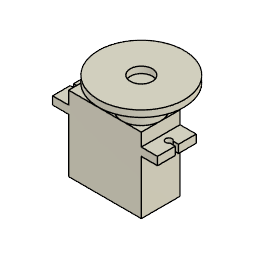
Enclosure (Autodesk Fusion 360 archive; units mm, degrees)
design "Servo"
Autodesk Fusion 360 part; units mm, degrees
sketch "Sketch1" plane through (0, 0, 0) normal (0, 0, 1) x (1, 0, 0)
  line L0 (0, 0) -> (22.5, 0)
  line L1 (22.5, 23.2) -> (0, 23.2)
  line L2 (22.5, 23.2) -> (22.5, 19.2)
  line L3 (22.5, 19.2) -> (27.5, 19.2)
  line L4 (27.5, 19.2) -> (27.5, 16.7)
  line L5 (27.5, 16.7) -> (22.5, 16.7)
  line L6 (0, 23.2) -> (0, 19.2)
  line L7 (0, 19.2) -> (-5, 19.2)
  line L8 (-5, 19.2) -> (-5, 16.7)
  line L9 (-5, 16.7) -> (0, 16.7)
  line L10 (22.5, 0) -> (22.5, 16.7)
  line L11 (22.5, 19.2) -> (22.5, 23.2)
  line L12 (0, 23.2) -> (0, 19.2)
  line L13 (0, 16.7) -> (0, 0)
  dimension "d1" = 22.5
  dimension "d2" = 23.2
  dimension "d3" = 4
  dimension "d4" = 5
  dimension "d5" = 2.5
  dimension "d6" = 4
  dimension "d7" = 5
  dimension "d8" = 2.5
  constraint coincident L0.start L13.end
  constraint horizontal L0
  constraint perpendicular L0 L10
  constraint perpendicular L1 L11
  constraint perpendicular L0 L13
  constraint perpendicular L1 L2
  constraint perpendicular L2 L3
  constraint perpendicular L3 L4
  constraint perpendicular L5 L10
  constraint perpendicular L1 L6
  constraint perpendicular L6 L7
  constraint perpendicular L7 L8
  constraint perpendicular L9 L13
  constraint collinear L10 L11
  constraint collinear L12 L13
  measures "d1" distance of L0.start L0.end
  measures "d2" distance of L0.end L1.start
  measures "d3" distance of L1.start L2.end
  measures "d4" distance of L2.end L3.end
  measures "d5" distance of L3.end L4.end
  measures "d6" distance of L1.end L6.end
  measures "d7" distance of L6.end L7.end
  measures "d8" distance of L7.end L8.end
extrude "Extrude1" add sketch "Sketch1" along normal blind 12
move_body "Move1" bodies 1 to x (1, 0, 0) y (0, 0, 1) z (0, -1, 0) at (0, 35.2, 8.8)
sketch "Sketch2" plane through (0, 0, 28) normal (0, 0, 1) x (-1, 0, 0)
  line L0 (-27.5, -35.2) -> (-22.5, -35.2)
  line L1 (-22.5, -35.2) -> (-22.5, -23.2)
  line L2 (-22.5, -23.2) -> (-27.5, -23.2)
  line L3 (-27.5, -23.2) -> (-27.5, -35.2)
  line L4 (-27.5, -29.2) -> (-27.5, -29.7)
  line L5 (-27.5, -29.2) -> (-27.5, -28.7)
  line L6 (-27.5, -29.7) -> (-25.866, -29.7)
  line L7 (-27.5, -28.7) -> (-25.866, -28.7)
  arc A0 (-25.866, -29.7) -> (-25.866, -28.7) centre (-25, -29.2) ccw
  dimension "d11" = 2
  dimension "d12" = 0.5
  dimension "d13" = 0.5
  constraint midpoint L3 L4.start
  constraint coincident L3 L4.end
  constraint coincident L3 L5.end
  constraint perpendicular L4 L6
  constraint perpendicular L5 L7
  measures "d11" diameter of A0
  measures "d12" distance of L4.start L4.end
  measures "d13" distance of L4.start L5.end
extrude "Extrude2" cut sketch "Sketch2" against normal blind 7 contours L3 L4 L5 L6 L7 A0
sketch "Sketch3" plane through (0, 0, 28) normal (0, 0, 1) x (-1, 0, 0)
  line L0 (0, -35.2) -> (5, -35.2)
  line L1 (5, -35.2) -> (5, -23.2)
  line L2 (5, -23.2) -> (0, -23.2)
  line L3 (0, -23.2) -> (0, -35.2)
  line L4 (0, -29.2) -> (1.5, -29.2)
  line L5 (5, -29.2) -> (5, -29.7)
  line L6 (5, -29.2) -> (5, -28.7)
  line L7 (5, -29.7) -> (3.366, -29.7)
  line L8 (5, -28.7) -> (3.366, -28.7)
  arc A0 (3.366, -28.7) -> (3.366, -29.7) centre (2.5, -29.2) ccw
  dimension "d16" = 1.5
  dimension "d17" = 2
  dimension "d18" = 0.5
  dimension "d19" = 0.5
  constraint midpoint L3 L4.start
  constraint perpendicular L3 L4
  constraint coincident L4.end A0
  constraint midpoint L1 L5.start
  constraint coincident L1 L5.end
  constraint coincident L1 L6.end
  constraint perpendicular L1 L7
  constraint perpendicular L6 L8
  measures "d16" distance of L4.start L4.end
  measures "d17" diameter of A0
  measures "d18" distance of L5.start L5.end
  measures "d19" distance of L5.start L6.end
extrude "Extrude3" cut sketch "Sketch3" against normal blind 18 contours L1 L5 L6 L7 L8 A0
sketch "Sketch4" plane through (0, 0, 32) normal (0, 0, 1) x (-1, 0, 0)
  line L0 (-22.5, -35.2) -> (0, -35.2)
  line L1 (0, -35.2) -> (0, -23.2)
  line L2 (0, -23.2) -> (-22.5, -23.2)
  line L3 (-22.5, -23.2) -> (-22.5, -35.2)
  arc A0 (-11.1636, -31.9427) -> (-11.1636, -26.4573) centre (-10.6, -29.2) ccw
  arc A1 (-11.1636, -26.4573) -> (-11.1636, -31.9427) centre (-16.5, -29.2) ccw
  dimension "d24" = 5.6
  constraint tangent L2 A1
  measures "d24" diameter of A0
extrude "Extrude4" add sketch "Sketch4" along normal blind 4.4 contours A0 A1
sketch "Sketch5" plane through (0, 0, 36.4) normal (0, 0, 1) x (-1, 0, 0)
  arc A0 (-11.1636, -26.4573) -> (-11.1636, -31.9427) centre (-16.5, -29.2) ccw
  arc A1 (-11.1636, -31.9427) -> (-11.1636, -26.4573) centre (-10.6, -29.2) ccw
  circle A2 centre (-16.5, -29.2) radius 2.4
  dimension "d27" = 4.8
  constraint concentric A0 A2
  measures "d27" diameter of A2
extrude "Extrude5" add sketch "Sketch5" along normal blind 2.9 contours A2
sketch "Sketch6" plane through (0, 0, 39.3) normal (0, 0, 1) x (-1, 0, 0)
  circle A0 centre (-16.5, -29.2) radius 2.4
  circle A1 centre (-16.5, -29.2) radius 3.4
  dimension "d30" = 6.8
  constraint concentric A0 A1
  measures "d30" diameter of A1
extrude "Extrude6" add sketch "Sketch6" against normal blind 1.8
sketch "Sketch7" plane through (0, 0, 39.3) normal (0, 0, 1) x (-1, 0, 0)
  circle A0 centre (-16.5, -29.2) radius 3.4
  circle A1 centre (-16.5, -29.2) radius 13.25
  dimension "d33" = 26.5
  constraint concentric A0 A1
  measures "d33" diameter of A1
extrude "Extrude7" add sketch "Sketch7" along normal blind 2

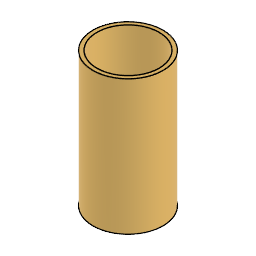
design "9mm Round"
Autodesk Fusion 360 part; units mm, degrees
sketch "Sketch1" plane through (0, 0, 0) normal (0, 0, 1) x (1, 0, 0)
  circle A0 centre (0, 0) radius 4.93
  dimension "d1" = 9.86
  constraint coincident A0.centre origin
  measures "d1" diameter of A0
extrude "Extrude1" add sketch "Sketch1" along normal blind 3
sketch "Sketch2" plane through (0, 0, 3) normal (0, 0, 1) x (-1, 0, 0)
  circle A0 centre (0, 0) radius 4.93
  circle A1 centre (0, 0) radius 4.38
  dimension "d4" = -0.55
extrude "Extrude2" add sketch "Sketch2" along normal blind 15.95

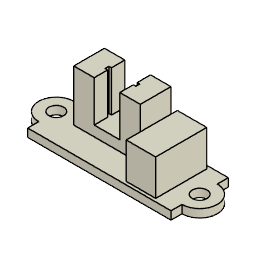
design "Photo Interruptor"
Autodesk Fusion 360 part; units mm, degrees
sketch "Sketch1" plane through (0, 0, 0) normal (0, 0, 1) x (1, 0, 0)
  line L0 (0, 13.8) -> (28, 13.8)
  line L1 (28, 25) -> (0, 25)
  arc A0 (0, 22.85) -> (0, 15.95) centre (0, 19.4) ccw
  arc A1 (28, 15.95) -> (28, 22.85) centre (28, 19.4) ccw
  line L2 (28, 13.8) -> (28, 15.95)
  line L3 (28, 22.85) -> (28, 25)
  line L4 (0, 25) -> (0, 22.85)
  line L5 (0, 15.95) -> (0, 13.8)
  dimension "d1" = 11.2
  dimension "d2" = 28
  dimension "d3" = 6.9
  dimension "d4" = 6.9
  constraint vertical L4
  constraint perpendicular L0 L5
  constraint perpendicular L0 L2
  constraint perpendicular L1 L3
  constraint collinear L2 L3
  constraint coincident A1.centre L2
  constraint collinear L4 L5
  constraint coincident A0.centre L4
  measures "d1" distance of L1.end L0.start
  measures "d2" distance of L0.start L0.end
  measures "d3" diameter of A1
  measures "d4" diameter of A0
extrude "Extrude1" add sketch "Sketch1" along normal blind 1.6
sketch "Sketch2" plane through (0, 0, 1.6) normal (0, 0, 1) x (-1, 0, 0)
  line L0 (0, -15.95) -> (0, -13.8)
  line L1 (0, -13.8) -> (-28, -13.8)
  line L2 (-28, -13.8) -> (-28, -15.95)
  arc A0 (-28, -15.95) -> (-28, -22.85) centre (-28, -19.4) ccw
  line L3 (-28, -22.85) -> (-28, -25)
  line L4 (-28, -25) -> (0, -25)
  line L5 (0, -25) -> (0, -22.85)
  arc A1 (0, -22.85) -> (0, -15.95) centre (0, -19.4) ccw
  circle A2 centre (0, -19.4) radius 1.45
  circle A3 centre (-28, -19.4) radius 1.45
  dimension "d7" = 2.9
  dimension "d8" = 2.9
  constraint concentric A1 A2
  constraint concentric A0 A3
  measures "d7" diameter of A2
  measures "d8" diameter of A3
extrude "Extrude2" cut sketch "Sketch2" against normal blind 5 contours A2 | A3
sketch "Sketch3" plane through (0, 0, 1.6) normal (0, 0, 1) x (-1, 0, 0)
  circle A0 centre (-28, -19.4) radius 1.45
  circle A1 centre (0, -19.4) radius 1.45
  line L0 (0, -15.95) -> (0, -13.8)
  line L1 (0, -13.8) -> (-28, -13.8)
  line L2 (-28, -13.8) -> (-28, -15.95)
  arc A2 (-28, -15.95) -> (-28, -22.85) centre (-28, -19.4) ccw
  line L3 (-28, -22.85) -> (-28, -25)
  line L4 (-28, -25) -> (0, -25)
  line L5 (0, -25) -> (0, -22.85)
  arc A3 (0, -22.85) -> (0, -15.95) centre (0, -19.4) ccw
  line L6 (-28, -25) -> (-24.4, -25)
  line L7 (-24.4, -25) -> (-24.4, -24.4)
  line L8 (-24.4, -24.4) -> (-18.65, -24.4)
  line L9 (-18.65, -24.4) -> (-18.65, -14.4)
  line L10 (-18.65, -14.4) -> (-24.4, -14.4)
  line L11 (-24.4, -14.4) -> (-24.4, -24.4)
  dimension "d11" = 3.6
  dimension "d12" = 0.6
  dimension "d13" = 5.75
  dimension "d14" = 10
  constraint coincident L3.end L4.start
  constraint coincident L4 L6.end
  constraint perpendicular L4 L7
  constraint horizontal L8
  constraint vertical L9
  constraint horizontal L10
  constraint vertical L11
  measures "d11" distance of L3.end L6.end
  measures "d12" distance of L6.end L7.end
  measures "d13" distance of L7.end L8.end
  measures "d14" distance of L7.end L10.end
extrude "Extrude3" add sketch "Sketch3" along normal blind 7 contours L8 L9 L10 L11
sketch "Sketch4" plane through (0, 0, 1.6) normal (0, 0, 1) x (-1, 0, 0)
  line L0 (-24.4, -14.4) -> (-18.65, -14.4)
  line L1 (-18.65, -14.4) -> (-18.65, -24.4)
  line L2 (-18.65, -24.4) -> (-24.4, -24.4)
  line L3 (-24.4, -24.4) -> (-24.4, -14.4)
  circle A0 centre (-28, -19.4) radius 1.45
  circle A1 centre (0, -19.4) radius 1.45
  line L4 (0, -15.95) -> (0, -13.8)
  line L5 (0, -13.8) -> (-28, -13.8)
  line L6 (-28, -13.8) -> (-28, -15.95)
  arc A2 (-28, -15.95) -> (-28, -22.85) centre (-28, -19.4) ccw
  line L7 (-28, -22.85) -> (-28, -25)
  line L8 (-28, -25) -> (0, -25)
  line L9 (0, -25) -> (0, -22.85)
  arc A3 (0, -22.85) -> (0, -15.95) centre (0, -19.4) ccw
  line L10 (0, -25) -> (-4, -25)
  line L11 (-4, -25) -> (-17, -25)
  line L12 (-4, -25) -> (-4, -19)
  line L13 (-4, -19) -> (-4, -18.8)
  line L14 (-4, -18.8) -> (-17, -18.8)
  line L15 (-17, -18.8) -> (-17, -24.8)
  line L16 (-17, -24.8) -> (-4, -24.8)
  line L17 (-4, -24.8) -> (-4, -18.8)
  dimension "d17" = 4
  dimension "d18" = 13
  dimension "d19" = 6
  dimension "d20" = 0.2
  dimension "d21" = 13
  dimension "d22" = 6
  constraint coincident L8.end L9.start
  constraint coincident L8 L10.end
  constraint coincident L8 L11.end
  constraint perpendicular L8 L12
  constraint vertical L13
  constraint horizontal L14
  constraint vertical L15
  constraint horizontal L16
  constraint vertical L17
  measures "d17" distance of L8.end L10.end
  measures "d18" distance of L10.end L11.end
  measures "d19" distance of L10.end L12.end
  measures "d20" distance of L12.end L13.end
  measures "d21" distance of L13.end L14.end
  measures "d22" distance of L13.end L16.end
extrude "Extrude4" add sketch "Sketch4" along normal blind 2 contours L12 L13 L14 L15 L16 L17
sketch "Sketch5" plane through (0, 0, 3.6) normal (0, 0, 1) x (-1, 0, 0)
  line L0 (-4, -24.8) -> (-4, -18.8)
  line L1 (-4, -18.8) -> (-17, -18.8)
  line L2 (-17, -18.8) -> (-17, -24.8)
  line L3 (-17, -24.8) -> (-4, -24.8)
  line L4 (-4, -24.8) -> (-8, -24.8)
  line L5 (-8, -24.8) -> (-8, -18.8)
  line L6 (-8, -18.8) -> (-4, -18.8)
  line L7 (-4, -18.8) -> (-4, -24.8)
  line L8 (-17, -24.8) -> (-13, -24.8)
  line L9 (-13, -24.8) -> (-13, -18.8)
  line L10 (-13, -18.8) -> (-17, -18.8)
  line L11 (-17, -18.8) -> (-17, -24.8)
  dimension "d25" = 4
  dimension "d26" = 4
  constraint horizontal L4
  constraint vertical L5
  constraint horizontal L6
  constraint vertical L7
  constraint coincident L0.start L3.end
  constraint horizontal L8
  constraint vertical L9
  constraint horizontal L10
  constraint vertical L11
  constraint coincident L2.end L3.start
  measures "d25" distance of L0.start L4.end
  measures "d26" distance of L2.end L8.end
extrude "Extrude5" add sketch "Sketch5" along normal blind 8 contours L0 L1 L3 L4 L5 L6 L7 | L1 L2 L3 L8 L9 L10 L11
sketch "Sketch6" plane through (8, 0, 0) normal (1, 0, 0) x (0, 1, 0)
  line L0 (18.8, 3.6) -> (24.8, 3.6)
  line L1 (24.8, 3.6) -> (24.8, 11.6)
  line L2 (24.8, 11.6) -> (18.8, 11.6)
  line L3 (18.8, 11.6) -> (18.8, 3.6)
  line L4 (21.8, 3.6) -> (21.8, 11.6)
  line L5 (21.8, 11.6) -> (21.425, 11.6)
  line L6 (21.8, 11.6) -> (22.175, 11.6)
  line L7 (21.425, 11.6) -> (22.175, 11.6)
  line L8 (22.175, 11.6) -> (22.175, 3.6)
  line L9 (22.175, 3.6) -> (21.425, 3.6)
  line L10 (21.425, 3.6) -> (21.425, 11.6)
  dimension "d29" = 0.375
  dimension "d30" = 0.375
  constraint midpoint L0 L4.start
  constraint midpoint L2 L4.end
  constraint coincident L2 L5.end
  constraint coincident L2 L6.end
  constraint horizontal L7
  constraint vertical L8
  constraint horizontal L9
  constraint vertical L10
  constraint coincident L0 L8.end
  measures "d29" distance of L4.end L5.end
  measures "d30" distance of L4.end L6.end
extrude "Extrude6" cut sketch "Sketch6" against normal blind 0.5 contours L0 L2 L4 L5 L7 L9 L10 | L0 L2 L4 L6 L7 L8 L9
sketch "Sketch7" plane through (13, 0, 0) normal (-1, 0, 0) x (0, -1, 0)
  line L0 (-24.8, 3.6) -> (-18.8, 3.6)
  line L1 (-18.8, 3.6) -> (-18.8, 11.6)
  line L2 (-18.8, 11.6) -> (-24.8, 11.6)
  line L3 (-24.8, 11.6) -> (-24.8, 3.6)
  line L4 (-21.8, 11.6) -> (-22.175, 11.6)
  line L5 (-21.8, 11.6) -> (-21.425, 11.6)
  line L6 (-22.175, 11.6) -> (-21.425, 11.6)
  line L7 (-21.425, 11.6) -> (-21.425, 3.6)
  line L8 (-21.425, 3.6) -> (-22.175, 3.6)
  line L9 (-22.175, 3.6) -> (-22.175, 11.6)
  dimension "d33" = 0.375
  dimension "d34" = 0.375
  constraint midpoint L2 L4.start
  constraint coincident L2 L4.end
  constraint coincident L2 L5.end
  constraint horizontal L6
  constraint vertical L7
  constraint horizontal L8
  constraint vertical L9
  constraint coincident L0 L7.end
  measures "d33" distance of L4.start L4.end
  measures "d34" distance of L4.start L5.end
extrude "Extrude7" cut sketch "Sketch7" against normal blind 0.5 contours L0 L2 L4 L5 L6 L7 L8 L9

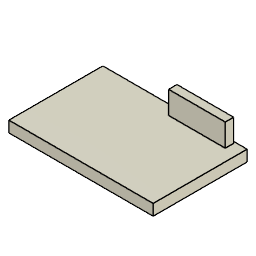
design "Display"
Autodesk Fusion 360 part; units mm, degrees
sketch "Sketch1" plane through (0, 0, 0) normal (0, 0, 1) x (1, 0, 0)
  line L0 (0, 0) -> (-85.5, 0)
  line L1 (-85.5, 0) -> (-85.5, 55.7)
  line L2 (-85.5, 55.7) -> (0, 55.7)
  line L3 (0, 55.7) -> (0, 0)
  dimension "d1" = 85.5
  dimension "d2" = 55.7
  constraint horizontal L0
  constraint vertical L1
  constraint horizontal L2
  constraint vertical L3
  constraint coincident L0.start L3.end
  measures "d1" distance of L0.start L0.end
  measures "d2" distance of L0.start L2.end
extrude "Extrude1" add sketch "Sketch1" along normal blind 6.6 makes body 1
sketch "Sketch2" plane through (0, 0, 6.6) normal (0, 0, 1) x (-1, 0, 0)
  line L0 (0, -55.7) -> (85.5, -55.7)
  line L1 (85.5, -55.7) -> (85.5, 0)
  line L2 (85.5, 0) -> (0, 0)
  line L3 (0, 0) -> (0, -55.7)
  line L4 (0, -5) -> (7, -5)
  line L5 (7, 0) -> (7, -1)
  line L6 (7, -1) -> (40.6, -1)
  line L7 (40.6, -1) -> (40.6, -6)
  line L8 (40.6, -6) -> (7, -6)
  line L9 (7, -6) -> (7, -1)
  dimension "d5" = 7
  dimension "d6" = 1
  dimension "d7" = 33.6
  dimension "d8" = 5
  constraint coincident L3 L4.start
  constraint perpendicular L3 L4
  constraint coincident L2 L5.start
  constraint perpendicular L2 L5
  constraint horizontal L6
  constraint vertical L7
  constraint horizontal L8
  constraint vertical L9
  measures "d5" distance of L4.start L4.end
  measures "d6" distance of L5.start L5.end
  measures "d7" distance of L5.end L6.end
  measures "d8" distance of L5.end L8.end
extrude "Extrude2" add sketch "Sketch2" along normal blind 13.4 contours L6 L7 L8 L9 bodies 1
mirror "Mirror1" about plane through (-85.5, 55.7, 0) normal (0, 1, 0) of bodies 1 makes body 2
delete_body "RemoveBody1" bodies 1
move_body "Move1" bodies 2 to x (1, 0, 0) y (0, 1, 0) z (0, 0, 1) at (0, -56, 0)

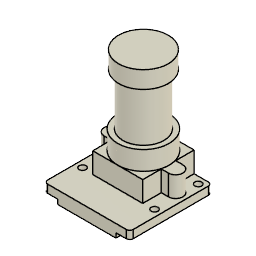
design "Camera"
Autodesk Fusion 360 part; units mm, degrees
sketch "Sketch1" plane through (0, 0, 0) normal (0, 0, 1) x (1, 0, 0)
  line L0 (0, 0) -> (25, 0)
  line L1 (25, 0) -> (25, -24)
  line L2 (25, -24) -> (0, -24)
  line L3 (0, -24) -> (0, 0)
  dimension "d1" = 25
  dimension "d2" = 24
  constraint horizontal L0
  constraint vertical L1
  constraint horizontal L2
  constraint vertical L3
  constraint coincident L0.start L3.end
  measures "d1" distance of L0.start L0.end
  measures "d2" distance of L0.start L2.end
extrude "Extrude1" add sketch "Sketch1" along normal blind 1.6
sketch "Sketch2" plane through (0, 0, 1.6) normal (0, 0, 1) x (-1, 0, 0)
  line L0 (0, 24) -> (-25, 24)
  line L1 (-25, 24) -> (-25, 0)
  line L2 (-25, 0) -> (0, 0)
  line L3 (0, 0) -> (0, 24)
  line L4 (-12.5, 0) -> (-4, 0)
  line L5 (-12.5, 0) -> (-21, 0)
  line L6 (-4, 0) -> (-4, 5)
  line L7 (-4, 5) -> (-21, 5)
  line L8 (-21, 5) -> (-21, 0)
  dimension "d5" = 8.5
  dimension "d6" = 8.5
  dimension "d7" = 5
  constraint midpoint L2 L4.start
  constraint parallel L2 L4
  constraint parallel L2 L5
  constraint perpendicular L4 L6
  constraint perpendicular L6 L7
  constraint perpendicular L2 L8
  measures "d5" distance of L4.start L4.end
  measures "d6" distance of L4.start L5.end
  measures "d7" distance of L4.end L6.end
extrude "Extrude2" add sketch "Sketch2" along normal blind 2.1 contours L2 L4 L5 L6 L7 L8
extrude "Extrude3" add 1 faces at (15.3333, -17.6667, 1.6) along direction (0, 0, 1) blind 0.75
move_body "Move1" bodies 1 to x (1, 0, 0) y (0, -1, 0) z (0, 0, -1) at (0, -24, 4.7)
sketch "Sketch3" plane through (0, 0, 4.7) normal (0, 0, 1) x (-1, 0, 0)
  line L0 (-25, 0) -> (0, 0)
  line L1 (0, 0) -> (0, 24)
  line L2 (0, 24) -> (-25, 24)
  line L3 (-25, 24) -> (-25, 0)
  line L4 (-12.5, 0) -> (-19.8, 0)
  line L5 (-12.5, 0) -> (-5.2, 0)
  line L6 (-5.2, 15) -> (-19.8, 15)
  line L7 (-19.8, 5.4) -> (-21.9, 5.4)
  line L8 (-19.8, 9.6) -> (-21.9, 9.6)
  line L9 (-5.2, 5.4) -> (-3.1, 5.4)
  line L10 (-5.2, 9.6) -> (-3.1, 9.6)
  arc A0 (-3.1, 5.4) -> (-3.1, 9.6) centre (-3.1, 7.5) ccw
  line L11 (-5.2, 0) -> (-5.2, 5.4)
  line L12 (-5.2, 9.6) -> (-5.2, 15)
  arc A1 (-21.9, 9.6) -> (-21.9, 5.4) centre (-21.9, 7.5) ccw
  line L13 (-19.8, 15) -> (-19.8, 9.6)
  line L14 (-19.8, 5.4) -> (-19.8, 0)
  dimension "d12" = 7.3
  dimension "d13" = 7.3
  dimension "d14" = 15
  dimension "d21" = 4.2
  dimension "d22" = 4.2
  constraint midpoint L0 L4.start
  constraint parallel L0 L4
  constraint parallel L0 L5
  constraint perpendicular L0 L11
  constraint perpendicular L6 L12
  constraint perpendicular L4 L14
  constraint tangent L7 A1
  constraint tangent L8 A1
  constraint tangent L9 A0
  constraint tangent L10 A0
  constraint collinear L11 L12
  constraint collinear L13 L14
  measures "d12" distance of L4.start L4.end
  measures "d13" distance of L4.start L5.end
  measures "d14" distance of L5.end L6.start
  measures "d21" diameter of A0
  measures "d22" diameter of A1
extrude "Extrude4" add sketch "Sketch3" along normal blind 6 contours L0 L4 L5 L6 L7 L8 L9 L10 A0 L11 L12 A1 L13 L14
sketch "Sketch4" plane through (0, 0, 10.7) normal (0, 0, 1) x (-1, 0, 0)
  line L0 (-5.2, 9.6) -> (-5.2, 15)
  line L1 (-5.2, 15) -> (-19.8, 15)
  line L2 (-19.8, 15) -> (-19.8, 9.6)
  line L3 (-19.8, 9.6) -> (-21.9, 9.6)
  arc A0 (-21.9, 9.6) -> (-21.9, 5.4) centre (-21.9, 7.5) ccw
  line L4 (-21.9, 5.4) -> (-19.8, 5.4)
  line L5 (-19.8, 5.4) -> (-19.8, 0)
  line L6 (-19.8, 0) -> (-5.2, 0)
  line L7 (-5.2, 0) -> (-5.2, 5.4)
  line L8 (-5.2, 5.4) -> (-3.1, 5.4)
  arc A1 (-3.1, 5.4) -> (-3.1, 9.6) centre (-3.1, 7.5) ccw
  line L9 (-3.1, 9.6) -> (-5.2, 9.6)
  circle A2 centre (-12.5, 7.5) radius 7.5
extrude "Extrude5" add sketch "Sketch4" along normal blind 5.5 contours A2
sketch "Sketch5" plane through (0, 0, 16.2) normal (0, 0, 1) x (-1, 0, 0)
  circle A0 centre (-12.5, 7.5) radius 7.5
  circle A1 centre (-12.5, 7.5) radius 6
  dimension "d27" = 12
  constraint concentric A0 A1
  measures "d27" diameter of A1
extrude "Extrude6" add sketch "Sketch5" along normal blind 20 contours A1
sketch "Sketch6" plane through (0, 0, 36.2) normal (0, 0, 1) x (-1, 0, 0)
  circle A0 centre (-12.5, 7.5) radius 6
  circle A1 centre (-12.5, 7.5) radius 7.25
  dimension "d30" = 14.5
  constraint concentric A0 A1
  measures "d30" diameter of A1
extrude "Extrude7" add sketch "Sketch6" against normal blind 5
sketch "Sketch7" plane through (0, 0, 2.35) normal (0, 0, -1) x (1, 0, 0)
  line L0 (4, 19) -> (4, 24)
  line L1 (4, 24) -> (0, 24)
  line L2 (0, 24) -> (0, 0)
  line L3 (0, 0) -> (25, 0)
  line L4 (25, 0) -> (25, 24)
  line L5 (25, 24) -> (21, 24)
  line L6 (21, 24) -> (21, 19)
  line L7 (21, 19) -> (4, 19)
  line L8 (0, 0) -> (2, 0)
  line L9 (2, 0) -> (2, 2)
  circle A0 centre (2, 2) radius 1
  line L10 (25, 0) -> (23, 0)
  line L11 (23, 0) -> (23, 2)
  circle A1 centre (23, 2) radius 1
  line L12 (25, 0) -> (25, 14.75)
  line L13 (25, 14.75) -> (23, 14.75)
  line L14 (0, 0) -> (0, 14.75)
  line L15 (0, 14.75) -> (2, 14.75)
  circle A2 centre (2, 14.75) radius 1
  circle A3 centre (23, 14.75) radius 1
  dimension "d35" = 2
  dimension "d36" = 2
  dimension "d37" = 2
  dimension "d38" = 2
  dimension "d39" = 2
  dimension "d40" = 2
  dimension "d41" = 14.75
  dimension "d42" = 2
  dimension "d43" = 14.75
  dimension "d44" = 2
  dimension "d45" = 2
  dimension "d46" = 2
  constraint coincident L2.end L3.start
  constraint coincident L3 L8.end
  constraint perpendicular L8 L9
  constraint coincident L9.end A0.centre
  constraint coincident L3.end L4.start
  constraint coincident L3 L10.end
  constraint perpendicular L3 L11
  constraint coincident L11.end A1.centre
  constraint coincident L4 L12.end
  constraint perpendicular L4 L13
  constraint coincident L2 L14.end
  constraint perpendicular L14 L15
  constraint coincident L15.end A2.centre
  constraint coincident L13.end A3.centre
  measures "d35" distance of L2.end L8.end
  measures "d36" distance of L8.end L9.end
  measures "d37" diameter of A0
  measures "d38" distance of L3.end L10.end
  measures "d39" distance of L10.end L11.end
  measures "d40" diameter of A1
  measures "d41" distance of L3.end L12.end
  measures "d42" distance of L12.end L13.end
  measures "d43" distance of L2.end L14.end
  measures "d44" distance of L14.end L15.end
  measures "d45" diameter of A2
  measures "d46" diameter of A3
fillet "Fillet1" radius 1 4 edges at (0, 0, 3.525) (0, -24, 3.525) (25, 0, 3.525) (25, -24, 3.525)
extrude "Extrude8" cut sketch "Sketch7" against normal blind 10 contours A0 | A1 | A2 | A3

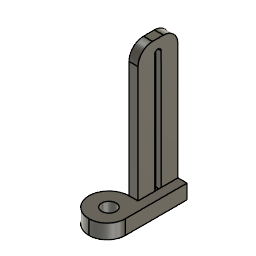
design "Photo Sensor Mount"
Autodesk Fusion 360 part; units mm, degrees
sketch "Sketch1" plane through (0, 0, 0) normal (0, 0, 1) x (1, 0, 0)
  circle A0 centre (0, 0) radius 2
  line L0 (-0.0705, 5.4995) -> (6.9295, 5.4995)
  line L1 (6.9295, 5.4995) -> (6.9295, -5.4995)
  line L2 (6.9295, -5.4995) -> (0.0716, -5.4995)
  arc A1 (-0.0705, 5.4995) -> (0.0716, -5.4995) centre (0, 0) ccw
  dimension "d1" = 4
  dimension "d3" = 7
  dimension "d4" = 11
  constraint coincident A0.centre A1.centre
  constraint horizontal L0
  constraint vertical L1
  constraint horizontal L2
  constraint concentric A0 A1
  measures "d1" diameter of A0
  measures "d3" distance of L0.start L0.end
  measures "d4" distance of L0.start L2.end
extrude "Extrude1" add sketch "Sketch1" along normal blind 4 makes body 1
sketch "Sketch2" plane through (0, 0, 4) normal (0, 0, 1) x (-1, 0, 0)
  circle A0 centre (0, 0) radius 2
  line L0 (-6.9295, -5.4995) -> (0.0705, -5.4995)
  arc A1 (0.0705, -5.4995) -> (-0.0716, 5.4995) centre (0, 0) ccw
  line L1 (-0.0716, 5.4995) -> (-6.9295, 5.4995)
  line L2 (-6.9295, 5.4995) -> (-6.9295, -5.4995)
  line L3 (-6.9295, -5.4995) -> (-2.4295, -5.4995)
  line L4 (-2.4295, -5.4995) -> (-2.4295, 5.4995)
  line L5 (-2.4295, 5.4995) -> (-6.9295, 5.4995)
  line L6 (-6.9295, 5.4995) -> (-6.9295, -5.4995)
  dimension "d7" = 4.5
  constraint horizontal L3
  constraint vertical L4
  constraint horizontal L5
  constraint vertical L6
  constraint coincident L1 L4.end
  constraint coincident L0.start L2.end
  measures "d7" distance of L0.start L3.end
extrude "Extrude2" add sketch "Sketch2" along normal blind 36 contours L0 L1 L2 L3 L4 L5 L6 bodies 1
sketch "Sketch3" plane through (0, -5.4995, 0) normal (0, -1, 0) x (1, 0, 0)
  line L0 (0.0716, 0) -> (6.9295, 0)
  line L1 (6.9295, 0) -> (6.9295, 40)
  line L2 (6.9295, 40) -> (2.4295, 40)
  line L3 (2.4295, 40) -> (2.4295, 4)
  line L4 (2.4295, 4) -> (0.0716, 4)
  line L5 (0.0716, 4) -> (0.0716, 0)
  line L6 (0.0716, 4) -> (2.4295, 9.5549)
  line L7 (0.0716, 4) -> (6.1062, 4) construction
  dimension "d10" = 67
  constraint horizontal L7
  constraint coincident L4.end L5.start
  constraint coincident L3 L6.end
  measures "d10" angle of L6 L7
extrude "Extrude3" add sketch "Sketch3" against normal blind 1 contours L3 L4 L6 bodies 1
sketch "Sketch4" plane through (0, 5.4995, 0) normal (0, 1, 0) x (-1, 0, 0)
  line L0 (-6.9295, 0) -> (0.0705, 0)
  line L1 (0.0705, 0) -> (0.0705, 4)
  line L2 (0.0705, 4) -> (-2.4295, 4)
  line L3 (-2.4295, 4) -> (-2.4295, 40)
  line L4 (-2.4295, 40) -> (-6.9295, 40)
  line L5 (-6.9295, 40) -> (-6.9295, 0)
  line L6 (0.0705, 4) -> (-2.4295, 9.8896)
  line L7 (0.0705, 4) -> (6.4687, 4) construction
  dimension "d13" = 113
  constraint horizontal L7
  constraint coincident L1.end L2.start
  constraint coincident L3 L6.end
  measures "d13" angle of L6 L7
extrude "Extrude4" add sketch "Sketch4" against normal blind 1 contours L2 L3 L6 bodies 1
sketch "Sketch5" plane through (6.9295, 0, 0) normal (1, 0, 0) x (0, 1, 0)
  line L0 (-5.4995, 0) -> (5.4995, 0)
  line L1 (5.4995, 0) -> (5.4995, 40)
  line L2 (5.4995, 40) -> (-5.4995, 40)
  line L3 (-5.4995, 40) -> (-5.4995, 0)
  line L4 (0, 2) -> (0.0035, 2)
  line L5 (0.0035, 2) -> (0, 2)
  line L6 (0, 38) -> (0.0292, 38)
  line L7 (1.3, 36.8608) -> (1.3, 3.307)
  arc A0 (1.3, 36.8608) -> (-1.3, 36.5855) centre (0.0146, 36.5855) ccw
  line L8 (-1.3, 3.4017) -> (-1.3, 36.5855)
  arc A1 (-1.3, 3.4017) -> (1.3, 3.307) centre (0.0017, 3.4017) ccw
  dimension "d17" = 2
  constraint horizontal L5
  constraint horizontal L6
  measures "d17" distance of origin L4.start
extrude "Extrude5" cut sketch "Sketch5" against normal blind 4 contours L7 A0 L8 A1 bodies 1
extrude "Extrude6" cut 1 faces at (6.9295, -4.0997, 25.5285) along direction (-1, 0, 0) blind 2 on bodies 1 bodies 1
sketch "Sketch6" plane through (2.9295, 0, 0) normal (1, 0, 0) x (0, 1, 0)
  arc A0 (1.3, 36.8608) -> (-1.3, 36.5855) centre (0.0146, 36.5855) ccw
  line L0 (-1.3, 36.5855) -> (-1.3, 3.4017)
  arc A1 (-1.3, 3.4017) -> (1.3, 3.307) centre (0.0017, 3.4017) ccw
  line L1 (1.3, 3.307) -> (1.3, 36.8608)
  line L2 (-0.8604, 36.5855) -> (-0.8733, 3.4021)
  line L3 (0.8767, 3.4017) -> (0.8896, 36.5852)
  arc A2 (0.8896, 36.5852) -> (-0.8604, 36.5855) centre (0.0146, 36.5855) ccw
  arc A3 (-0.8733, 3.4021) -> (0.8767, 3.4017) centre (0.0017, 3.4017) ccw
  dimension "d25" = 1.75
  dimension "d26" = 1.75
  constraint concentric A0 A2
  constraint concentric A1 A3
  constraint tangent L2 A3
  constraint tangent L3 A2
  constraint parallel L2 L3
  measures "d25" diameter of A2
  measures "d26" diameter of A3
extrude "Extrude7" cut sketch "Sketch6" against normal blind 1 contours L2 L3 A2 A3 bodies 1
extrude "Extrude8" add 1 faces at (2.9295, -1.0112, 25.5244) along direction (1, 0, 0) blind 1 on bodies 1 bodies 1
fillet "Fillet1" radius 4 2 edges at (3.6795, -5.4995, 40) (3.6795, 5.4995, 40) on bodies 1
sketch "Sketch7" plane through (0, 0, 0) normal (0, 0, 1) x (1, 0, 0)
  circle A0 centre (0, 19) radius 2
  line L0 (0, 24.5) -> (5, 24.5)
  line L1 (0, 13.5) -> (0, 8.5)
  line L2 (5, 24.5) -> (5, 8.5)
  line L3 (5, 8.5) -> (0, 8.5)
  arc A1 (0, 24.5) -> (0, 13.5) centre (0, 19) ccw
  dimension "d33" = 4
  dimension "d35" = 5
  constraint tangent L0 A1
  constraint perpendicular L0 L2
  constraint perpendicular L1 L3
  constraint concentric A0 A1
  measures "d33" diameter of A0
  measures "d35" distance of L1.start L1.end
extrude "Extrude9" add sketch "Sketch7" along normal blind 4 separate body makes body 2
move_body "Move1" bodies 1 to x (1, 0, 0) y (0, 1, 0) z (0, 0, 1) at (0, -8.9863, 0.4962)
extrude "Extrude10" add 1 faces at (3.3333, 8.5, 1.3333) along direction (0, -1, 0) blind 5 on bodies 2 bodies 2
fillet "Fillet2" radius 5 1 edges at (5, 24.5, 2) on bodies 2
mirror "Mirror1" about plane through (0, 0, 0) normal (0, 1, 0) of bodies 2 makes body 3
move_body "Move2" bodies 3 to x (1, 0, 0) y (0, 1, 0) z (0, 0, 1) at (0, -16, 0)
extrude "Extrude11" add 1 faces at (3.3333, -19.5, 1.3333) along direction (0, 1, 0) blind 1 on bodies 3 bodies 3
move_body "Move3" bodies 1 to x (-1, 0, 0) y (0, -1, 0) z (0, 0, 1) at (4.859, -22.9545, 0)
move_body "Move4" bodies 1 to x (1, 0, 0) y (0, 1, 0) z (0, 0, 1) at (0, 3, 0)
split "Split1" by plane through (2.4295, -16.4677, 4.4962) normal (1, 0, 0) bodies 1 makes body 4 at (5.3354, -5.4888, 1.8295)
move_body "Move5" bodies 1 to x (1, 0, 0) y (0, 1, 0) z (0, 0, 1) at (0, -13, -0.5)
move_body "Move6" bodies 1 to x (1, 0, 0) y (0, 1, 0) z (0, 0, 1) at (6.8, 0, 0)
extrude "Extrude12" cut 1 faces at (3.3333, -18.5, 1.3333) along direction (0, -1, 0) blind 11 on bodies 3 bodies 3
move_body "Move7" bodies 1 to x (1, 0, 0) y (0, 1, 0) z (0, 0, 1) at (-6.7, 0, 0)
move_body "Move8" bodies 1 to x (1, 0, 0) y (0, 1, 0) z (0, 0, 1) at (0, -0.0323, 0)
move_body "Move9" bodies 1 to x (1, 0, 0) y (0, 1, 0) z (0, 0, 1) at (-0.0295, 0, 0)
combine "Combine1" operation add target body 1 tool bodies 3
extrude "Extrude13" add 1 faces at (4.1667, -29.5, 1.3333) along direction (0, 1, 0) blind 11 on bodies 1 bodies 1
delete_body "RemoveBody1" bodies 2
delete_body "RemoveBody2" bodies 4
